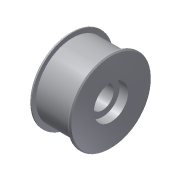
# Autodesk Inventor part: Wheel
Saved by Autodesk Inventor 2014 SP1 (Build 180222100, 222)
## iProperties
Created: 2014-04-22
Part Number: Wheel
Material: Aluminum 6061
Document SubType Name: Modeling
Designer: Rauhul Varma
Density: 2.71 g/cm^3
Appearance: Aluminum - Flat
Mass: 136.552 g
Surface Area: 124.961 cm^2
Volume: 50.3882 cm^3
Author: Rauhul Varma
Autodesk Inventor part; units mm, degrees
ref_plane "YZ Plane" through (0, 0, 0) normal (1, 0, 0) x (0, 1, 0)
ref_plane "XZ Plane" through (0, 0, 0) normal (0, 1, 0) x (-1, 0, 0)
ref_plane "XY Plane" through (0, 0, 0) normal (0, 0, 1) x (1, 0, 0)
sketch "Sketch1" plane through (0, 0, 0) normal (0, 0, 1) x (1, 0, 0)
  line L0 (0, 0) -> (0, 7.9375) construction
  line L1 (0, 25.4) -> (12.7, 25.4)
  line L2 (12.7, 25.4) -> (12.7, 28.575)
  line L3 (12.7, 28.575) -> (14.2875, 28.575)
  line L4 (14.2875, 28.575) -> (14.2875, 12)
  line L5 (14.2875, 12) -> (8.2875, 12)
  line L6 (8.2875, 12) -> (8.2875, 7.9375)
  line L7 (8.2875, 7.9375) -> (0, 7.9375)
  line L8 (0, 0) -> (14.2875, 0) construction
  line L9 (14.2875, 0) -> (14.2875, 12) construction
  line L10 (0, 7.9375) -> (0, 25.4)
  dimension "d3" = 25.4
  dimension "d4" = 28.575
  dimension "d5" = 12
  dimension "d6" = 7.9375
  dimension "d7" = 6
  dimension "d8" = 14.2875
  dimension "d9" = 1.5875
  constraints: 22 end point, 10 parallel, 3 perpendicular, 2 vertical, 1 coincident
  measures "d3" distance from line of point (0, 0) L1
  measures "d4" distance from line of point (0, 0) L3
  measures "d5" distance from line of point (0, 0) L5
  measures "d6" distance from line of point (0, 0) L7
  measures "d7" distance of L4.end L5.end
  measures "d8" distance between parallel lines of L0 L4
  measures "d9" distance between parallel lines of L4 L2
revolve "Revolution1" add sketch "Sketch1" angle 360 about axis through (0, 0, 0) along (1, 0, 0)
mirror "Mirror1" about plane through (0, 25.4, 0) normal (-1, 0, 0)
sketch "Sketch2" plane through (-14.2875, 0, 0) normal (-1, 0, 0) x (0, 0, 1)
  circle A0 centre (0, 0) radius 12 projected
  circle A1 centre (0, 0) radius 28.575 projected
  circle A2 centre (0, 0) radius 15.875 construction
  line L0 (0, 0) -> (0, 15.875) construction
  circle A3 centre (0, 15.875) radius 2.54 construction
  circle A4 centre (-13.7482, -7.9375) radius 2.54 construction
  circle A5 centre (13.7482, -7.9375) radius 2.54 construction
  circle A6 centre (0, 0) radius 20.6375
  point P0 (0, 13.335)
  point P1 (0, 12)
  dimension "d11" = 5.08
  dimension "d27" = 31.75
  dimension "d15" = 360
  dimension "d28" = 5.08
  dimension "d29" = 5.08
  dimension "d40" = 41.275
  constraints: 6 coincident, 3 centre point, 3 vertical alignment, 2 end point, 2 point on line, 1 vertical, 9 other
  measures "d28" diameter of A4
  measures "d29" diameter of A5
  measures "d40" diameter of A6
chamfer "Chamfer1" distance 0.7937 angle 45 2 edges at (-14.2875, -28.575, 0) (14.2875, -28.575, 0)
extrude "Extrusion2" add sketch "Sketch2" along normal blind 0.7937 contours A6
sketch "Sketch4" plane through (-15.0812, 0, 0) normal (-1, 0, 0) x (0, 0, 1)
  point P0 (0, 15.875)
  point P1 (-13.7482, -7.9375)
  point P2 (13.7482, -7.9375)
hole "Hole3" at (-15.0812, -7.9375, 13.7482) at (-15.0812, -7.9375, -13.7482) at (-15.0813, 15.875, 0) direction (1, 0, 0) diameter 3.302 depth 12.7 tip angle 118 thread size "8-32 UNC" class "2B" standard "ANSI Unified Screw Threads"
body "Solid2"
